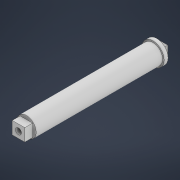
# Autodesk Inventor part: Verbindung_Rocker_Body
Saved by Autodesk Inventor 2021 (Build 250183000, 183)
## iProperties
Created: 2021-01-29
Part Number: Verbindung_Rocker_Body
Material: Generisch
Document SubType Name: Modeling
Designer: Ctroi
Density: 1 g/cm^3
Appearance: Vorgabe
Author: Ctroi
Autodesk Inventor part; units mm, degrees
ref_plane "YZ Plane" through (0, 0, 0) normal (1, 0, 0) x (0, 1, 0)
ref_plane "XZ Plane" through (0, 0, 0) normal (0, 1, 0) x (-1, 0, 0)
ref_plane "XY Plane" through (0, 0, 0) normal (0, 0, 1) x (1, 0, 0)
sketch "Skizze1" plane through (0, 0, 0) normal (0, 0, 1) x (1, 0, 0)
  line L0 (-4.75, 4.75) -> (4.75, 4.75)
  line L1 (4.75, 4.75) -> (4.75, -4.75)
  line L2 (4.75, -4.75) -> (-4.75, -4.75)
  line L3 (-4.75, -4.75) -> (-4.75, 4.75)
  line L4 (-4.75, 4.75) -> (4.75, -4.75) construction
  line L5 (4.75, 4.75) -> (-4.75, -4.75) construction
  point P0 (0, 0)
  dimension "d0" = 9.5
  dimension "d1" = 9.5
  constraints: 12 end point, 2 midpoint, 2 parallel, 1 horizontal, 1 perpendicular
  measures "d0" distance of L1.end L2.end
  measures "d1" distance of L0.end L1.end
extrude "Extrusion1" add sketch "Skizze1" along normal blind 3.5
sketch "Skizze2" plane through (0, 0, 3.5) normal (0, 0, 1) x (1, 0, 0)
  circle A0 centre (0, 0) radius 8.5
  dimension "d4" = 17
  constraints: 1 centre point, 1 coincident
  measures "d4" diameter of A0
extrude "Extrusion2" add sketch "Skizze2" along normal blind 3
sketch "Skizze3" plane through (0, 0, 6.5) normal (0, 0, 1) x (1, 0, 0)
  circle A0 centre (0, 0) radius 7.4
  circle A1 centre (0, 0) radius 8.5 projected
  dimension "d7" = 14.8
  dimension "d19" = 1.1
  constraints: 1 centre point
  measures "d7" diameter of A0
  measures "d19" radial gap between concentric circles of A1 A0
extrude "Extrusion3" add sketch "Skizze3" along normal blind 96 contours A0
sketch "Skizze4" plane through (0, 0, 102.5) normal (0, 0, 1) x (1, 0, 0)
  line L0 (-4.75, -4.75) -> (4.75, -4.75) projected
  line L1 (-4.75, 4.75) -> (4.75, 4.75)
  line L2 (4.75, 4.75) -> (4.75, -4.75)
  line L3 (4.75, -4.75) -> (-4.75, -4.75)
  line L4 (-4.75, -4.75) -> (-4.75, 4.75)
  line L5 (-4.75, 4.75) -> (4.75, -4.75) construction
  line L6 (4.75, 4.75) -> (-4.75, -4.75) construction
  point P0 (0, 0)
  dimension "d10" = 9.5
  constraints: 12 end point, 2 midpoint, 2 parallel, 1 horizontal, 1 perpendicular
  measures "d10" distance of L0.end L3.end
extrude "Extrusion4" add sketch "Skizze4" along normal blind 6
sketch "Skizze5" plane through (0, 0, 108.5) normal (0, 0, 1) x (1, 0, 0)
  circle A0 centre (0, 0) radius 2.25
  dimension "d13" = 4.5
  constraints: 1 centre point, 1 coincident
  measures "d13" diameter of A0
extrude "Extrusion5" cut sketch "Skizze5" against normal blind 5
sketch "Skizze6" plane through (0, 0, 0) normal (0, 0, -1) x (-1, 0, 0)
  circle A0 centre (0, 0) radius 2.25
  dimension "d16" = 4.5
  constraints: 1 centre point, 1 coincident
  measures "d16" diameter of A0
extrude "Extrusion6" cut sketch "Skizze6" against normal blind 5
